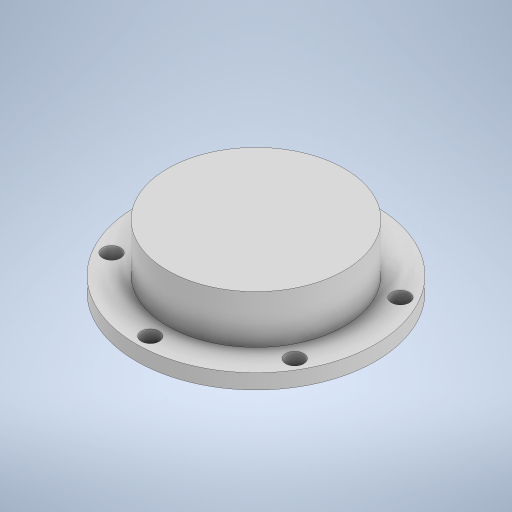
# Autodesk Inventor part: Module_bottom_Icicles26
Saved by Autodesk Inventor 2023 (Build 270158000, 158)
## iProperties
Created: 2022-10-30
Part Number: Module_bottom_Icicles26
Material: Generic
Document SubType Name: Modeling
Designer: incep
Density: 1 g/cm^3
Appearance: Default
Author: incep
Autodesk Inventor part; units mm, degrees
ref_plane "YZ Plane" through (0, 0, 0) normal (1, 0, 0) x (0, 1, 0)
ref_plane "XZ Plane" through (0, 0, 0) normal (0, 1, 0) x (-1, 0, 0)
ref_plane "XY Plane" through (0, 0, 0) normal (0, 0, 1) x (1, 0, 0)
sketch "Sketch1" plane through (0, 0, 0) normal (0, 1, 0) x (-1, 0, 0)
  circle A0 centre (0, 0) radius 24
  circle A1 centre (0, 0) radius 21.25 construction
  circle A2 centre (0, -21.25) radius 1.8
  circle A3 centre (18.403, -10.625) radius 1.8
  circle A4 centre (18.403, 10.625) radius 1.8
  circle A5 centre (0, 21.25) radius 1.8
  circle A6 centre (-18.403, 10.625) radius 1.8
  circle A7 centre (-18.403, -10.625) radius 1.8
  dimension "d9" = 42.5
  dimension "d7" = 48
  dimension "d11" = 3.6
  dimension "d22" = 360
  constraints: 7 centre point, 2 coincident, 1 vertical alignment, 15 other
  measures "d7" diameter of A0
  measures "d11" diameter of A2
extrude "Extrusion1" add sketch "Sketch1" along normal blind 3
sketch "Sketch2" plane through (0, 3, 0) normal (0, 1, 0) x (1, 0, 0)
  circle A0 centre (0, 0) radius 17.75
  dimension "d26" = 35.5
  constraints: 1 centre point, 1 coincident
  measures "d26" diameter of A0
extrude "Extrusion3" add sketch "Sketch2" along normal blind 9.7
equation "\"d9\" = iciclesMountD"
equation "\"d7\" = iciclesBaseOuterD"
equation "\"d11\" = clearanceM6"
equation "\"d24\" = isiclesBaseThickness"
equation "\"d26\" = iciclesPlugD"
equation "\"d30\" = chairThickness - isiclesBaseThickness"
equation "\"moduleHeight\" = 96"
equation "\"moduleMountD\" = 6.8"
equation "\"moduleCornerR\" = 5"
equation "\"d4\" = moduleCornerR"
equation "\"d5\" = moduleMountD"
equation "\"d6\" = moduleMountD"
equation "\"d8\" = moduleMountD"
equation "\"d10\" = moduleMountD"
equation "\"moduleOpeningR\" = 25"
equation "\"d13\" = moduleOpeningR"
equation "\"thickness\" = 6"
equation "\"d15\" = thickness"
equation "\"d16\" = 0"
equation "\"iciclesMountD\" = 42.5"
equation "\"d17\" = iciclesMountD"
equation "\"clearanceM6\" = 3.6"
equation "\"d18\" = clearanceM6"
equation "\"d21\" = 360deg"
equation "\"d0\" = moduleHeight"
equation "\"iciclesBaseOuterD\" = 48"
equation "\"iciclesPlugD\" = 35.5"
equation "\"chairThickness\" = 12.7"
equation "\"isiclesBaseThickness\" = 3"
body "Solid1"
